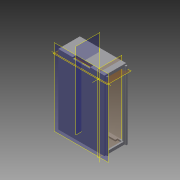
# Autodesk Inventor part: PI_Skal_med_rals
Saved by Autodesk Inventor 2015 (Build 190159000, 159)
## iProperties
Created: 2015-11-29
Part Number: PI_Skal_med_rals
Material: Generic
Document SubType Name: Modeling
Designer: abberik
Density: 1 g/cm^3
Appearance: Default
Author: abberik
Autodesk Inventor part; units mm, degrees
sketch "Sketch1" plane through (0, 0, 0) normal (0, 1, 0) x (-1, 0, 0)
  point P0 (0, 0)
sketch "Sketch2" plane through (0, 0, 0) normal (0, 1, 0) x (-1, 0, 0)
  circle A0 centre (0, 0) radius 1.25
  line L0 (60.55, 0) -> (-11.55, 0) projected
  line L1 (0, -71.35) -> (0, 13.35) projected
  circle A1 centre (49, 0) radius 1.25
  circle A2 centre (0, -58) radius 1.25
  circle A3 centre (49, -58) radius 1.25
  dimension "d0" = 2.5
  dimension "d3" = 49
  dimension "d6" = 58
  constraints: 4 centre point, 1 coincident, 1 horizontal, 1 vertical, 6 other
  measures "d0" diameter of A0
  measures "d3" distance of A0.centre A1.centre
  measures "d6" distance of A0.centre A2.centre
extrude "Extrusion1" add sketch "Sketch2" along normal blind 10
sketch "Sketch3" plane through (0, 0, 0) normal (0, 1, 0) x (-1, 0, 0)
  line L0 (52.5, 3.5) -> (-3.5, 3.5)
  line L1 (-3.5, 3.5) -> (-3.5, -85)
  line L2 (-3.5, -85) -> (52.5, -85)
  line L3 (52.5, -85) -> (52.5, 3.5)
  circle A0 centre (49, 0) radius 1.25 projected
  circle A1 centre (49, -58) radius 1.25 projected
  circle A2 centre (0, 0) radius 1.25 projected
  circle A3 centre (0, -58) radius 1.25 projected
  line L4 (54.5, 5.5) -> (-5.5, 5.5)
  line L5 (-5.5, 5.5) -> (-5.5, -87)
  line L6 (-5.5, -87) -> (54.5, -87)
  line L7 (54.5, -87) -> (54.5, 5.5)
  dimension "d11" = 3.5
  dimension "d12" = 27
  dimension "d13" = 3.5
  dimension "d14" = 3.5
  dimension "d15" = 2
  constraints: 16 end point, 4 parallel, 2 perpendicular, 1 horizontal, 3 other
  measures "d11" distance from line of L0 A0.centre
  measures "d12" distance from line of L2 A1.centre
  measures "d13" distance from line of L3 A0.centre
  measures "d14" distance from line of L1 A2.centre
  measures "d15" distance between parallel lines of L1 L5
extrude "Extrusion2" add sketch "Sketch3" along normal blind 2 contours L3 L2 L1 L0 | L7 L6 L5 L4
sketch "Sketch4" plane through (0, 2, 0) normal (0, 1, 0) x (1, 0, 0)
  line L0 (-54.5, 87) -> (-54.5, -5.5) projected
  line L1 (-54.5, -5.5) -> (5.5, -5.5) projected
  line L2 (5.5, 87) -> (-54.5, 87) projected
  line L3 (5.5, -5.5) -> (5.5, 87) projected
  point P0 (0, 0)
sketch "Sketch5" plane through (0, 0, 0) normal (0, 0, 1) x (1, 0, 0)
  line L0 (-54.5, 0) -> (5.5, 0) projected
  line L1 (5.5, 0) -> (5.5, 2) projected
  line L2 (-54.5, 2) -> (5.5, 2) projected
  line L3 (-54.5, 0) -> (-54.5, 2) projected
  line L4 (5.5, 0) -> (7.5, 0)
  line L5 (7.5, 0) -> (7.5, 30)
  line L6 (7.5, 30) -> (5.5, 30)
  line L7 (5.5, 30) -> (5.5, 0)
  point P0 (0, 0)
  dimension "d18" = 2
  dimension "d19" = 30
  constraints: 8 end point, 2 parallel, 1 horizontal, 1 perpendicular
  measures "d18" distance of L5.end L6.end
  measures "d19" distance of L4.end L5.end
sketch3d "3D Sketch1"
sketch3d "3D Sketch2"
  line L0 (5.5, 2, -87) -> (5.5, 2, 5.5)
  line L1 (5.5, 2, 5.5) -> (-54.5, 2, 5.5)
  line L2 (-54.5, 2, 5.5) -> (-54.5, 2, -87)
sweep "Sweep2" add profiles "Sketch5" path "3D Sketch2" contours L1 L7 L6 L5 L4
sketch "Sketch6" plane through (7.5, 0, -87) normal (0, 0, -1) x (-1, 0, 0)
  line L0 (2, 30) -> (62, 30)
  line L1 (2, 30) -> (2, 2) projected
  line L2 (2, 25) -> (62, 25)
  line L3 (62, 30) -> (62, 2) projected
  line L4 (2, 25) -> (2, 2)
  line L5 (2, 2) -> (62, 2)
  line L6 (2, 2) -> (62, 2) projected
  line L7 (62, 25) -> (62, 2)
  line L8 (0, 0) -> (0, 30) projected
  line L9 (0, 30) -> (2, 30) projected
  line L10 (64, 0) -> (0, 0) projected
  line L11 (64, 0) -> (64, 30) projected
  line L12 (64, 30) -> (62, 30) projected
  point P0 (7.5, 0)
  dimension "d25" = 5
  constraints: 10 end point, 2 collinear, 2 horizontal, 2 point on line, 1 vertical
  measures "d25" distance between parallel lines of L2 L0
extrude "Extrusion3" add sketch "Sketch6" along normal blind 2 contours L0 L3 L2 L1 | L1 L5 L3 L12 L11 L10 L8 L9
sketch "Sketch8" plane through (-56.5, 30, 7.5) normal (0, 0, 1) x (1, 0, 0)
  line L0 (64, -30) -> (0, -30) projected
  line L1 (20, -30) -> (44, -30)
  line L2 (44, -30) -> (44, -25)
  line L3 (44, -25) -> (20, -25)
  line L4 (20, -25) -> (20, -30)
  line L5 (0, -30) -> (0, 0) projected
  line L6 (64, -30) -> (64, 0) projected
  point P0 (56.5, -30)
  dimension "d39" = 20
  dimension "d40" = 20
  dimension "d41" = 5
  constraints: 8 end point, 2 parallel, 1 horizontal, 1 perpendicular, 1 point on line
  measures "d39" distance between parallel lines of L5 L4
  measures "d40" distance between parallel lines of L6 L2
  measures "d41" distance between parallel lines of L0 L3
extrude "Extrusion5" cut sketch "Sketch8" against normal blind 2
sketch "Sketch9" plane through (0, 2, 0) normal (0, 1, 0) x (1, 0, 0)
  circle A0 centre (0, 0) radius 1.25 projected
  circle A1 centre (0, 0) radius 1.25 projected
  circle A2 centre (-49, 0) radius 1.25 projected
  circle A3 centre (-49, 0) radius 1.25 projected
  circle A4 centre (-49, 58) radius 1.25 projected
  circle A5 centre (-49, 58) radius 1.25 projected
  circle A6 centre (0, 58) radius 1.25 projected
  circle A7 centre (0, 58) radius 1.25 projected
  circle A8 centre (0, 58) radius 1.25 projected
  circle A9 centre (0, 0) radius 2.5
  circle A10 centre (-49, 0) radius 1.25 projected
  circle A11 centre (-49, 0) radius 2.5
  circle A12 centre (0, 58) radius 2.5
  circle A13 centre (-49, 58) radius 2.5
  dimension "d44" = 5
  dimension "d45" = 5
  dimension "d46" = 5
  dimension "d47" = 5
  constraints: 4 centre point, 4 coincident
  measures "d44" diameter of A9
  measures "d45" diameter of A11
  measures "d46" diameter of A12
  measures "d47" diameter of A13
extrude "Extrusion6" add sketch "Sketch9" along normal blind 4
sketch "Sketch12" plane through (7.5, 0, -89) normal (0, 0, -1) x (-1, 0, 0)
  line L0 (10, 6) -> (5, 6) projected
  line L1 (5, 2) -> (10, 2) projected
  line L2 (10, 6) -> (5, 6) projected
  line L3 (2, 30) -> (10, 30)
  line L4 (10, 30) -> (10, 28)
  line L5 (10, 28) -> (2, 28)
  line L6 (2, 28) -> (2, 30)
  line L7 (2, 25) -> (62, 25) projected
  line L8 (2, 28) -> (10, 28)
  line L9 (10, 28) -> (10, 25)
  line L10 (10, 25) -> (2, 25)
  line L11 (2, 25) -> (2, 28)
  point P0 (7.5, 0)
  dimension "d72" = 8
  dimension "d73" = 2
  constraints: 16 end point, 4 parallel, 2 horizontal, 2 perpendicular, 1 point on line
  measures "d72" distance of L4.end L5.end
  measures "d73" distance of L3.end L4.end
sketch "Sketch13" plane through (7.5, 0, 7.5) normal (1, 0, 0) x (0, 0, -1)
  line L0 (2, 5) -> (2, 2) projected
  line L1 (2, 30) -> (2, 2) projected
  line L2 (2, 30) -> (2, 2) projected
  line L3 (2, 2) -> (2, 5) projected
  line L4 (63, 2) -> (68, 2) projected
  line L5 (5, 2) -> (10, 2) projected
  line L6 (5, 2) -> (10, 2) projected
  line L7 (63, 2) -> (68, 2) projected
  line L8 (2, 2) -> (96.5, 2) projected
  line L9 (96.5, 2) -> (2, 2) projected
  line L10 (94.5, 25) -> (94.5, 30) projected
  line L11 (96.5, 25) -> (96.5, 2) projected
  line L12 (4, 26.5) -> (92.5, 26.5)
  line L13 (92.5, 26.5) -> (92.5, 4)
  line L14 (92.5, 4) -> (4, 4)
  line L15 (4, 4) -> (4, 26.5)
  line L16 (96.5, 30) -> (0, 30) projected
  line L17 (96.5, 2) -> (96.5, 25) projected
  point P0 (7.5, 0)
  dimension "d67" = 2
  dimension "d68" = 2
  dimension "d69" = 3.5
  dimension "d70" = 2
  constraints: 8 end point, 2 parallel, 1 horizontal, 1 perpendicular
  measures "d67" distance between parallel lines of L10 L13
  measures "d68" distance between parallel lines of L1 L15
  measures "d69" distance between parallel lines of L16 L12
  measures "d70" distance between parallel lines of L8 L14
extrude "Extrusion10" cut sketch "Sketch12" against normal up to surface (2 mm away) contours L5 L9 L7 L11
extrude "Extrusion11" cut sketch "Sketch13" against normal up to surface (2 mm away)
sketch "Sketch14" plane through (7.5, 0, -89) normal (0, 0, -1) x (-1, 0, 0)
  line L0 (64, 30) -> (66, 30)
  line L1 (66, 30) -> (66, 28)
  line L2 (66, 28) -> (64, 28)
  line L3 (64, 28) -> (64, 30)
  line L4 (66, 4) -> (64, 4)
  line L5 (64, 4) -> (64, 2)
  line L6 (64, 2) -> (66, 2)
  line L7 (66, 2) -> (66, 4)
  line L8 (64, 30) -> (0, 30) projected
  line L9 (64, 0) -> (64, 30) projected
  point P0 (7.5, 0)
  dimension "d78" = 2
  dimension "d79" = 2
  dimension "d80" = 2
  dimension "d81" = 2
  dimension "d82" = 0
  dimension "d83" = 0
  dimension "d84" = 0
  dimension "d85" = 24
  constraints: 16 end point, 4 parallel, 2 horizontal, 2 perpendicular
  measures "d78" distance of L1.end L2.end
  measures "d79" distance of L0.end L1.end
  measures "d80" distance of L6.end L5.end
  measures "d81" distance of L5.end L4.end
  measures "d82" distance between parallel lines of L8 L0
  measures "d83" distance between parallel lines of L9 L3
  measures "d84" distance between parallel lines of L9 L5
  measures "d85" distance between parallel lines of L2 L4
extrude "Extrusion12" add sketch "Sketch14" against normal blind 94.5
ref_plane "Work Plane1" through (-24.5, 0, 7.5) normal (-1, 0, 0) x (0, 0, 1)
mirror "Mirror1" about plane through (-24.5, 0, 7.5) normal (-1, 0, 0) of "Extrusion12"
sketch "Sketch15" plane through (-56.5, 0, 7.5) normal (-1, 0, 0) x (0, 0, 1)
  line L0 (-4, 4) -> (-92.5, 4) projected
  line L1 (-92.5, 26.5) -> (-4, 26.5) projected
  line L2 (-4, 26.5) -> (-4, 4) projected
  line L3 (-92.5, 4) -> (-92.5, 26.5) projected
  point P0 (-7.5, 0)
extrude "Extrusion13" cut sketch "Sketch15" against normal blind 2
body "Solid1"
